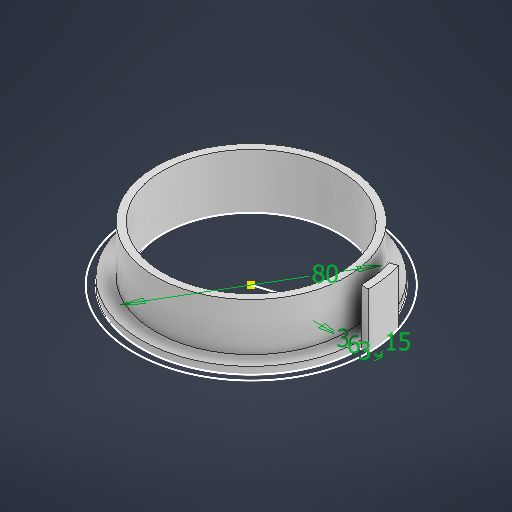
# Autodesk Inventor part: 80mm-CoilForm
Saved by Autodesk Inventor 2026 (Build 300175050, 175E)
## iProperties
Created: 2025-08-08
Part Number: 80mm-CoilForm
Material: Generic
Document SubType Name: Modeling
Designer: user
Density: 1 g/cm^3
Appearance: Default
Author: user
## iProperties of the stored document 80mm-CoilForm_3DPrint.ipt
Created: 2025-08-08
Part Number: 80mm-CoilForm_3DPrint
Material: Generic
Document SubType Name: Modeling
Designer: user
Density: 1 g/cm^3
Appearance: Default
Author: user
Autodesk Inventor part; units mm, degrees
ref_plane "YZ Plane" through (0, 0, 0) normal (1, 0, 0) x (0, 1, 0)
ref_plane "XZ Plane" through (0, 0, 0) normal (0, 1, 0) x (-1, 0, 0)
ref_plane "XY Plane" through (0, 0, 0) normal (0, 0, 1) x (1, 0, 0)
sketch "Sketch1" plane through (0, 0, 0) normal (0, 1, 0) x (-1, 0, 0)
  circle A0 centre (0, 0) radius 40
  circle A1 centre (0, 0) radius 46
  circle A2 centre (0, 0) radius 37
  circle A3 centre (0, 0) radius 49
  line L0 (-46, 0) -> (-49, 0)
  line L1 (0, 0) -> (-46.7041, -14.8233)
  point P0 (-43.8446, -13.9157)
  dimension "d0" = 80
  dimension "d1" = 6
  dimension "d2" = 3
  dimension "d7" = 3
  dimension "d8" = 15
  constraints: 4 end point, 3 centre point, 2 point on circle, 1 coincident, 1 horizontal, 1 horizontal alignment, 3 other
  measures "d0" diameter of A0
  measures "d2" radial gap between concentric circles of A0 A2
  measures "d8" distance of L0.end L1.end
extrude "Extrusion1" add sketch "Sketch1" along normal blind 23 contours A0
extrude "Extrusion2" add sketch "Sketch1" along normal blind 3 contours A1
extrude "Extrusion3" add sketch "Sketch1" along normal up to surface (23 mm away) contours L1 A3 L0 A1 picked at (-46.1746, -12.9028)
body "Solid1"
